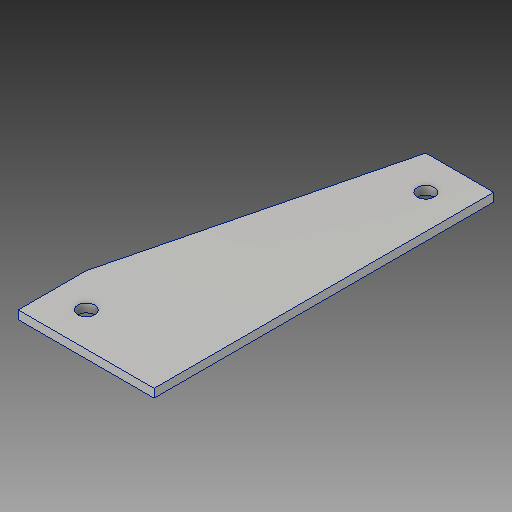
# Autodesk Inventor part: 15102898-16-P-0213
Saved by Autodesk Inventor 2017 (Build 210142000, 142)
## iProperties
Created: 2016-10-05
Part Number: 15102898-16-P-0213
Material: Aluminum 6061
Document SubType Name: Modeling
Designer: gus
Density: 2.7 g/cm^3
Appearance: Aluminum - Flat
Mass: 43.7021 g
Surface Area: 113.809 cm^2
Volume: 16.186 cm^3
Author: gus
Autodesk Inventor part; units mm, degrees
ref_plane "YZ Plane" through (0, 0, 0) normal (1, 0, 0) x (0, 1, 0)
ref_plane "XZ Plane" through (0, 0, 0) normal (0, 1, 0) x (-1, 0, 0)
ref_plane "XY Plane" through (0, 0, 0) normal (0, 0, 1) x (1, 0, 0)
sketch "Sketch1" plane through (0, 0, 0) normal (0, 1, 0) x (-1, 0, 0)
  line L0 (0, 0) -> (25.4, 0)
  line L1 (25.4, -127) -> (0, -127)
  line L2 (0, -127) -> (0, 0)
  circle A0 centre (38.1, -12.7) radius 3.175
  circle A1 centre (12.7, -114.3) radius 3.175
  line L3 (25.4, -127) -> (50.8, -25.4)
  line L4 (50.8, -25.4) -> (50.8, 0)
  line L5 (50.8, 0) -> (0, 0)
  dimension "d0" = 25.4
  dimension "d1" = 127
  dimension "d2" = 6.35
  dimension "d3" = 6.35
  dimension "d4" = 12.7
  dimension "d6" = 12.7
  dimension "d7" = 12.7
  dimension "d10" = 25.4
  dimension "d11" = 50.8
  dimension "d12" = 12.7
  constraints: 12 end point, 2 centre point, 1 collinear, 1 horizontal, 1 parallel, 1 vertical
  measures "d0" distance of L1.start L1.end
  measures "d1" distance of L0.end L1.start
  measures "d2" diameter of A0
  measures "d3" diameter of A1
  measures "d4" distance from line of L2 A1.centre
  measures "d6" distance from line of L1 A1.centre
  measures "d7" distance from line of L0 A0.centre
  measures "d10" distance of L3.end L4.end
  measures "d11" distance of L4.end L0.start
  measures "d12" distance from line of L4 A0.centre
extrude "Extrusion1" add sketch "Sketch1" along normal blind 3.175
body "Solid1"
